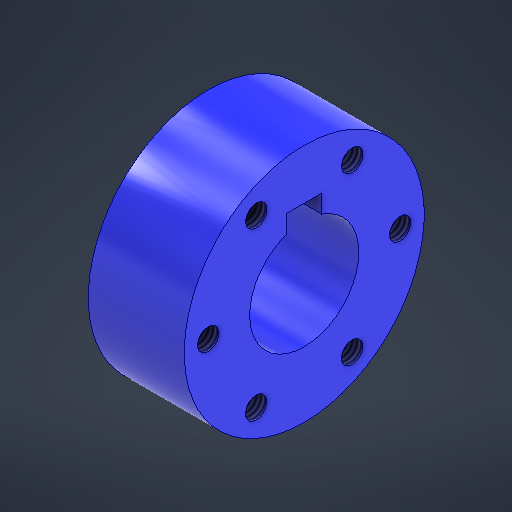
# Autodesk Inventor part: Befestigung bremsscheibe
Saved by Autodesk Inventor 2026.2 (Build 302298010, 298A)
## iProperties
Created: 2026-04-14
Part Number: Befestigung bremsscheibe
Material: Generisch
Document SubType Name: Modeling
Designer: pparr
Density: 1 g/cm^3
Appearance: Blau - Wandfarbe - glänzend
Author: pparr
Autodesk Inventor part; units mm, degrees
ref_plane "YZ Plane" through (0, 0, 0) normal (1, 0, 0) x (0, 1, 0)
ref_plane "XZ Plane" through (0, 0, 0) normal (0, 1, 0) x (-1, 0, 0)
ref_plane "XY Plane" through (0, 0, 0) normal (0, 0, 1) x (1, 0, 0)
sketch "Skizze1" plane through (0, 0, 0) normal (1, 0, 0) x (0, 1, 0)
  circle A0 centre (0, 0) radius 12.5
  circle A1 centre (0, 0) radius 16.25
  dimension "d0" = 25
  dimension "d1" = 32.5
  constraints: 2 centre point, 2 coincident
  measures "d0" diameter of A0
  measures "d1" diameter of A1
extrude "Extrusion1" add sketch "Skizze1" along normal mid plane 0.1
sketch "Skizze2" plane through (0.05, 0, 0) normal (1, 0, 0) x (0, 0, -1)
  circle A0 centre (0, 0) radius 27.5
  dimension "d5" = 55
  constraints: 1 centre point, 1 coincident
  measures "d5" diameter of A0
extrude "Extrusion2" add sketch "Skizze2" along normal blind 22
sketch "Skizze4" plane through (22.05, 0, 0) normal (1, 0, 0) x (0, 0, -1)
  circle A0 centre (0, 0) radius 12.5
  dimension "d8" = 25
  constraints: 1 centre point, 1 coincident
  measures "d8" diameter of A0
extrude "Extrusion3" cut sketch "Skizze4" against normal blind 30
sketch "Skizze5" plane through (0.05, 0, 0) normal (-1, 0, 0) x (0, 0, 1)
  point P0 (0, 0)
  point P1 (0.0333, -22)
  point P2 (19.0692, -10.9712)
  point P3 (19.0359, 11.0288)
  point P4 (-0.0333, 22)
  point P5 (-19.0692, 10.9712)
  point P6 (-19.0359, -11.0288)
  dimension "d18" = 22
  dimension "d21" = 360
  constraints: 7 other
  measures "d18" distance of point (0, 0) point (0.033, -22)
hole "Bohrung1" at (0.05, -22, 0.0333) at (0.05, -10.9712, 19.0692) at (0.05, 11.0288, 19.0359) at (0.05, 22, -0.0333) at (0.05, 10.9712, -19.0692) at (0.05, -11.0288, -19.0359) direction (1, 0, 0) diameter 4.917 end through all thread size "M6x1" class "6H" standard "ISO Metric profile"
sketch "Skizze6" plane through (22.05, 0, 0) normal (1, 0, 0) x (0, 0, -1)
  line L0 (-16, -4) -> (-9, -4)
  line L1 (-9, -4) -> (-9, 4)
  line L2 (-9, 4) -> (-16, 4)
  line L3 (-16, 4) -> (-16, -4)
  circle A0 centre (0, 0) radius 12.5 projected
  line L4 (-16, -4) -> (-9, 4) construction
  line L5 (-9, -4) -> (-16, 4) construction
  point P0 (-12.5, 0)
  point P1 (-11.8427, -4)
  point P2 (-11.8427, 4)
  dimension "d23" = 7
  dimension "d24" = 8
  dimension "d25" = 9
  constraints: 12 end point, 2 midpoint, 2 parallel, 1 horizontal, 1 perpendicular, 2 other
  measures "d23" distance of L2.end L1.end
  measures "d24" distance of L1.end L0.end
  measures "d25" distance from line of L1 point (0, 0)
extrude "Extrusion4" cut sketch "Skizze6" against normal blind 52 contours L3 L2 A0 L0
